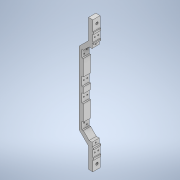
# Autodesk Inventor part: Axel_arch3
Saved by Autodesk Inventor 2020 (Build 240168000, 168)
## iProperties
Created: 2022-06-13
Part Number: Axel_arch3
Material: 일반
Document SubType Name: Modeling
Designer: samsung
Density: 1 g/cm^3
Appearance: 기본값
Author: samsung
Autodesk Inventor part; units mm, degrees
ref_plane "YZ Plane" through (0, 0, 0) normal (1, 0, 0) x (0, 1, 0)
sketch "스케치1" plane through (0, 0, 0) normal (0, 0, 1) x (1, 0, 0)
  line L0 (4.4817, -36) -> (19.4817, -36)
  line L1 (19.4817, 31.5) -> (22.4817, 31.5)
  line L2 (19.4817, 6.5) -> (22.4817, 6.5)
  line L3 (19.4817, 0) -> (22.4817, 0)
  line L4 (22.4817, 0) -> (22.4817, 6.5)
  line L5 (19.4817, 31.5) -> (19.4817, 6.5)
  line L6 (19.4817, 0) -> (19.4817, -36)
  line L7 (22.4817, 31.5) -> (19.4817, 31.5)
  line L8 (22.4817, 31.5) -> (22.4817, 36.5)
  line L9 (-13.5183, 152) -> (-18.5183, 152)
  line L10 (-18.5183, 152) -> (-18.5183, 182)
  line L11 (-18.5183, 182) -> (-13.5183, 182)
  line L12 (-13.5183, 96.5) -> (-18.5183, 96.5)
  line L13 (-18.5183, 96.5) -> (-18.5183, 71.5)
  line L14 (-18.5183, 71.5) -> (-13.5183, 71.5)
  line L15 (-28.5183, 192) -> (-13.5183, 192)
  line L16 (22.4817, 36.5) -> (16.4817, 36.5)
  line L17 (6.4817, 51.5) -> (-13.5183, 71.5)
  line L18 (4.4817, -36) -> (4.4817, 34)
  line L19 (-28.5183, 192) -> (-28.5183, 67)
  line L20 (4.4817, 34) -> (-28.5183, 67)
  line L21 (-13.5183, 96.5) -> (-13.5183, 152)
  line L22 (-13.5183, 182) -> (-13.5183, 192)
  line L23 (4.4817, 420) -> (19.4817, 420)
  line L24 (19.4817, 352.5) -> (22.4817, 352.5)
  line L25 (19.4817, 377.5) -> (22.4817, 377.5)
  line L26 (19.4817, 384) -> (22.4817, 384)
  line L27 (22.4817, 384) -> (22.4817, 377.5)
  line L28 (19.4817, 352.5) -> (19.4817, 377.5)
  line L29 (19.4817, 384) -> (19.4817, 420)
  line L30 (22.4817, 352.5) -> (19.4817, 352.5)
  line L31 (22.4817, 352.5) -> (22.4817, 347.5)
  line L32 (-13.5183, 232) -> (-18.5183, 232)
  line L33 (-18.5183, 232) -> (-18.5183, 202)
  line L34 (-18.5183, 202) -> (-13.5183, 202)
  line L35 (-13.5183, 287.5) -> (-18.5183, 287.5)
  line L36 (-18.5183, 287.5) -> (-18.5183, 312.5)
  line L37 (-18.5183, 312.5) -> (-13.5183, 312.5)
  line L38 (22.4817, 347.5) -> (16.4817, 347.5)
  line L39 (6.4817, 332.5) -> (-13.5183, 312.5)
  line L40 (4.4817, 420) -> (4.4817, 350)
  line L41 (-28.5183, 192) -> (-28.5183, 317)
  line L42 (4.4817, 350) -> (-28.5183, 317)
  line L43 (-13.5183, 287.5) -> (-13.5183, 232)
  line L44 (-13.5183, 202) -> (-13.5183, 192)
  line L45 (16.4817, 51.5) -> (6.4817, 51.5)
  line L46 (16.4817, 332.5) -> (6.4817, 332.5)
  line L47 (16.4817, 36.5) -> (16.4817, 51.5)
  line L48 (16.4817, 332.5) -> (16.4817, 347.5)
  dimension "d264" = 3
  dimension "d265" = 25
  dimension "d266" = 3
  dimension "d267" = 36
  dimension "d410" = 5
  dimension "d418" = 25
  dimension "d419" = 55.5
  dimension "d422" = 228
  dimension "d424" = 5
  dimension "d425" = 6
  dimension "d431" = 70
  dimension "d432" = 125
  dimension "d433" = 10
  dimension "d434" = 15
  dimension "d435" = 15
  dimension "d436" = 5
  constraints: 98 end point, 20 symmetric about line, 8 horizontal, 7 vertical, 6 perpendicular, 2 parallel
  measures "d264" distance of L2.start L2.end
  measures "d265" distance between parallel lines of L1 L2
  measures "d266" distance of L3.start L3.end
  measures "d267" distance between parallel lines of L0 L3
  measures "d410" distance of L10.end L11.end
  measures "d418" distance of L13.end L12.end
  measures "d419" distance between parallel lines of L9 L12
  measures "d422" distance between parallel lines of L15 L0
  measures "d424" distance of L1.end L8.end
  measures "d425" distance of L8.end L16.end
  measures "d431" distance of L0.start L18.end
  measures "d432" distance of L15.start L19.end
  measures "d433" distance of L11.end L15.end
  measures "d434" distance of L0.start L0.end
  measures "d435" distance of L15.start L15.end
  measures "d436" distance of L13.end L14.end
ref_plane "작업 평면1" through (0, 0, -63.413) normal (0, 0, -1) x (-1, 0, 0)
extrude "arch1" add sketch "스케치1" against normal blind 25
sketch "스케치23" plane through (-18.5183, 101.5, 0) normal (1, 0, 0) x (0, 0, -1)
  line L0 (0, 100.5) -> (0, 130.5) projected
  line L1 (25, 130.5) -> (25, 100.5) projected
  line L2 (25, 50.5) -> (25, 130.5)
  line L3 (25, 130.5) -> (0, 130.5)
  line L4 (0, 50.5) -> (25, 50.5)
  line L5 (0, 80.5) -> (25, 80.5)
  line L6 (0, 208.6982) -> (0, -27.6982) projected
  line L7 (25, -27.6982) -> (25, 208.6982) projected
  line L8 (0, 100.5) -> (25, 100.5)
  line L9 (0, 130.5) -> (0, 100.5)
  line L10 (0, 80.5) -> (0, 50.5)
  line L11 (0, 100.5) -> (25, 100.5) projected
  line L12 (0, 130.5) -> (25, 130.5) projected
  point P0 (0, -101.5)
  point P1 (0, 181)
  point P2 (0, 0)
  point P3 (25, 0)
  point P4 (25, 181)
  point P5 (12.5, 90.5)
  point P6 (6.5, 65.5)
  point P7 (18.5, 65.5)
  point P8 (6.5, 115.5)
  point P9 (18.5, 115.5)
  dimension "d285" = 25
  dimension "d286" = 30
  dimension "d290" = 30
  dimension "d291" = 6.5
  dimension "d292" = 6.5
  dimension "d293" = 6.5
  dimension "d294" = 6.5
  constraints: 14 end point, 3 parallel, 3 perpendicular, 3 point on line, 1 vertical
  measures "d285" distance of L3.end L2.end
  measures "d286" distance between parallel lines of L5 L4
  measures "d290" distance of L3.end L8.start
  measures "d291" distance from line of L10 point (6.5, 65.5)
  measures "d292" distance from line of L2 point (18.5, 65.5)
  measures "d293" distance from line of L9 point (6.5, 115.5)
  measures "d294" distance from line of L2 point (18.5, 115.5)
sketch "스케치24" plane through (19.4817, 6.5, 0) normal (1, 0, 0) x (0, 0, -1)
  line L0 (0, 0) -> (0, 25) projected
  line L1 (0, 0) -> (25, 0) projected
  line L2 (25, 25) -> (25, 0) projected
  line L3 (0, 346) -> (0, 371) projected
  line L4 (0, 346) -> (25, 346) projected
  line L5 (25, 371) -> (25, 346) projected
  line L6 (0, 371) -> (25, 371) projected
  line L7 (0, 25) -> (25, 25) projected
  point P0 (0, -6.5)
  point P1 (6.5, 12.5)
  point P2 (18.5, 12.5)
  point P3 (6.5, 358.5)
  point P4 (18.5, 358.5)
  dimension "d302" = 6.5
  dimension "d303" = 6.5
  dimension "d304" = 6.5
  dimension "d305" = 6.5
  measures "d302" distance from line of L0 point (6.5, 12.5)
  measures "d303" distance from line of L2 point (18.5, 12.5)
  measures "d304" distance from line of L3 point (6.5, 358.5)
  measures "d305" distance from line of L5 point (18.5, 358.5)
hole "구멍11" at (19.4817, 19, -6.5) at (19.4817, 19, -18.5) at (19.4817, 365, -6.5) at (19.4817, 365, -18.5) direction (-1, 0, 0) diameter 4.134 end through all thread size "M5x0.8" class "6H" standard "ISO Metric profile"
ref_plane "작업 평면5" through (22.4817, -36, 0) normal (1, 0, 0) x (0, 0, -1)
sketch "스케치27" plane through (22.4817, -36, 0) normal (1, 0, 0) x (0, 0, -1)
  line L0 (0, 420) -> (0, 457)
  line L1 (0, 457) -> (25, 457)
  line L2 (25, 36) -> (0, 36)
  line L3 (0, 36) -> (0, -1)
  line L4 (0, -1) -> (25, -1)
  line L5 (25, -1) -> (25, 36)
  line L6 (25, 457) -> (25, 420)
  line L7 (25, 388.5) -> (25, 456) projected
  line L8 (0, 420) -> (25, 420) projected
  line L9 (25, 420) -> (0, 420)
  point P0 (0, 36)
  point P1 (14, 438.5)
  point P2 (14, 17.5)
  dimension "d334" = 37
  dimension "d335" = 37
  dimension "d338" = 18.5
  dimension "d348" = 18.5
  dimension "d349" = 14
  dimension "d350" = 14
  constraints: 16 end point, 2 horizontal, 2 parallel, 2 point on line, 1 perpendicular
  measures "d334" distance of L0.start L0.end
  measures "d335" distance of L3.end L2.end
  measures "d338" distance from line of L2 point (14, 17.5)
  measures "d348" distance from line of point (14, 438.5) L8
  measures "d349" distance from line of L0 point (14, 438.5)
  measures "d350" distance from line of L3 point (14, 17.5)
hole "구멍12" at (22.4817, 402.5, -14) at (22.4817, -18.5, -14) direction (-1, 0, 0) diameter 8.376 end through all thread size "M10x1.5" class "6H" standard "ISO Metric profile"
hole "구멍14" at (-18.5183, 167, -6.5) at (-18.5183, 167, -18.5) at (-18.5183, 217, -6.5) at (-18.5183, 217, -18.5) direction (-1, 0, 0) diameter 4.134 end through all thread size "M5x0.8" class "6H" standard "ISO Metric profile"
sketch "스케치29" plane through (-28.5183, 67, 0) normal (-1, 0, 0) x (0, 0, 1)
  line L0 (0, 250) -> (0, 0) projected
  line L1 (0, 250) -> (-25, 250) projected
  line L2 (-25, 0) -> (-25, 250) projected
  line L3 (0, 0) -> (-25, 0) projected
  line L4 (0, 4.5) -> (-25, 4.5) projected
  line L5 (0, 29.5) -> (-25, 29.5) projected
  line L6 (0, 220.5) -> (-25, 220.5) projected
  line L7 (0, 245.5) -> (-25, 245.5) projected
  point P0 (0, -67)
  point P1 (-17, 12.5)
  point P2 (-8, 21.5)
  point P3 (-17, 237.5)
  point P4 (-8, 228.5)
  dimension "d438" = 8
  dimension "d439" = 8
  dimension "d440" = 8
  dimension "d441" = 8
  dimension "d442" = 8
  dimension "d443" = 8
  dimension "d444" = 8
  dimension "d459" = 8
  measures "d438" distance from line of L2 point (-17, 237.5)
  measures "d439" distance from line of L0 point (-8, 228.5)
  measures "d440" distance from line of L6 point (-8, 228.5)
  measures "d441" distance from line of L4 point (-17, 12.5)
  measures "d442" distance from line of L2 point (-17, 12.5)
  measures "d443" distance from line of L5 point (-8, 21.5)
  measures "d444" distance from line of L0 point (-8, 21.5)
  measures "d459" distance from line of point (-17, 237.5) L7
hole "구멍16" at (-28.5183, 79.5, -17) at (-28.5183, 88.5, -8) at (-28.5183, 304.5, -17) at (-28.5183, 295.5, -8) direction (1, 0, 0) diameter 4.134 end through all counterbore diameter 9 counterbore depth 5 thread size "M5x0.8" class "6H" standard "ISO Metric profile"
sketch "스케치31" plane through (16.4817, 36.5, 0) normal (1, 0, 0) x (0, 0, -1)
  line L0 (0, 0) -> (0, 15) projected
  line L1 (0, 0) -> (25, 0) projected
  line L2 (25, 15) -> (25, 0) projected
  line L3 (0, 15) -> (25, 15) projected
  line L4 (0, 296) -> (0, 311) projected
  line L5 (0, 296) -> (25, 296) projected
  line L6 (25, 311) -> (25, 296) projected
  line L7 (0, 311) -> (25, 311) projected
  point P0 (0, -36.5)
  point P1 (12.5, 7.5)
  point P2 (12.5, 303.5)
hole "구멍18" at (16.4817, 44, -12.5) at (16.4817, 340, -12.5) direction (-1, 0, 0) diameter 4.134 depth 10 tip angle 118 thread size "M5x0.8" class "6H" standard "ISO Metric profile"
